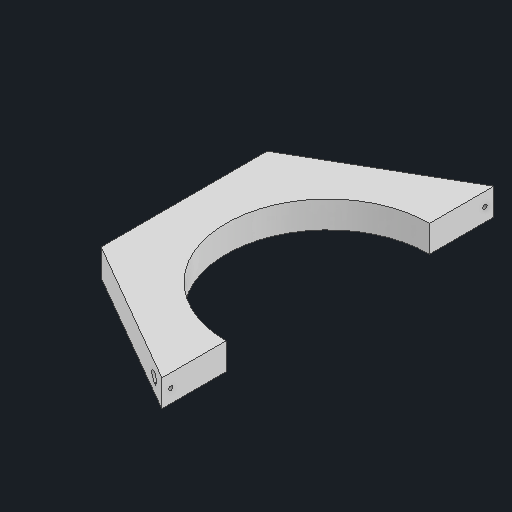
# Autodesk Inventor part: nowtrying_up
Saved by Autodesk Inventor 2026.3 (Build 303398000, 398)
## iProperties
Created: 2026-06-04
Part Number: nowtrying_up
Material: 一般
Document SubType Name: Modeling
Designer: shusu
Density: 1 g/cm^3
Appearance: 既定
Author: shusu
Autodesk Inventor part; units mm, degrees
sketch "スケッチ1" plane through (0, 0, 0) normal (0, 1, 0) x (-1, 0, 0)
  arc A0 (0, -57) -> (0, 57) centre (0, 0) ccw
  line L0 (0, 0) -> (80.5404, 46.5) construction
  line L1 (0, 0) -> (0, 93) construction
  line L2 (0, 93) -> (80.5404, 46.5)
  line L3 (80.5404, 46.5) -> (80.5404, 0)
  line L4 (80.5404, 0) -> (57, 0)
  line L5 (0, 0) -> (0, -93) construction
  line L6 (0, -93) -> (80.5404, -46.5)
  line L7 (80.5404, -46.5) -> (80.5404, 0)
  line L8 (0, -93) -> (0, -57)
  line L9 (0, 93) -> (0, 57)
  dimension "d0" = 57
  constraints: 20 end point, 3 point on circle, 2 coincident, 2 collinear, 2 symmetric about line, 1 centre point, 1 vertical
  measures "d0" radius of A0
extrude "押し出し1" add sketch "スケッチ1" along normal blind 15
sketch "スケッチ2" plane through (0, 0, 93) normal (1, 0, 0) x (0, 0, -1)
  line L0 (36, 0) -> (36, 15) projected
  line L1 (36, 15) -> (5, 15)
  line L2 (46.5, 15) -> (0, 15) projected
  line L3 (5, 15) -> (5, 7.5)
  line L4 (93, 0) -> (93, 15)
  line L5 (139.5, 15) -> (46.5, 15) projected
  line L6 (181, 15) -> (181, 7.5)
  dimension "d5" = 31
  dimension "d6" = 7.5
  constraints: 8 end point, 2 symmetric about line, 1 midpoint, 1 perpendicular, 1 point on line
  measures "d5" distance of L0.end L1.end
  measures "d6" distance of L1.end L3.end
hole "穴1" at (0, 7.5, 88) direction (-1, 0, 0) diameter 2.459 end through all thread size "M3x0.5" class "6H" standard "ISO Metric profile"
sketch "スケッチ3" plane through (0, 0, 93) normal (-0.5, 0, 0.866) x (0.866, 0, 0.5)
  ellipse E0 centre (-10, 7.5) end of major axis (-12.459, 7.5) minor radius 1.2295 projected
  point P0 (-46.5, 0)
  point P1 (-7.541, 7.5)
  constraints: 1 horizontal alignment, 1 other
sketch "スケッチ5" plane through (0, 0, 93) normal (-0.5, 0, 0.866) x (0.866, 0, 0.5)
  ellipse E0 centre (-10, 7.5) end of major axis (-12.459, 7.5) minor radius 1.2295 projected
  point P0 (-46.5, 0)
  point P1 (-12.459, 7.5)
  constraints: 1 horizontal alignment, 1 other
ref_plane "作業平面3" through (-8.6603, 7.5, 88) normal (0, 0, -1) x (-1, 0, 0)
sketch "スケッチ7" plane through (-8.6603, 7.5, 88) normal (0, 0, -1) x (-1, 0, 0)
  line L0 (0, 0) -> (4.8, 0)
  point P0 (-8.6603, -7.5)
  dimension "d21" = 4.8
  constraints: 2 end point, 1 horizontal
  measures "d21" distance of L0.start L0.end
ref_plane "作業平面4" through (-13.4603, 7.5, 88) normal (-1, 0, 0) x (0, 0, 1)
sketch "スケッチ8" plane through (-13.4603, 7.5, 88) normal (-1, 0, 0) x (0, 0, 1)
  point P0 (-88, -7.5)
  point P1 (0, 0)
hole "穴3" at (-13.4603, 7.5, 88) direction (1, 0, 0) diameter 2.459 end through all counterbore diameter 5.5 counterbore depth 5 thread size "M3x0.5" class "6H" standard "ISO Metric profile"
sketch "スケッチ9" plane through (0, 15, 0) normal (0, 1, 0) x (1, 0, 0)
  point P0 (0, 0)
  point P1 (0, 0)
  constraints: 1 coincident
ref_plane "作業平面5" through (0, 15, 0) normal (0, 0, 1) x (1, 0, 0)
hole "穴4" at (0, 7.5, -88) direction (-1, 0, 0) diameter 2.459 end through all thread size "M3x0.5" class "6H" standard "ISO Metric profile"
